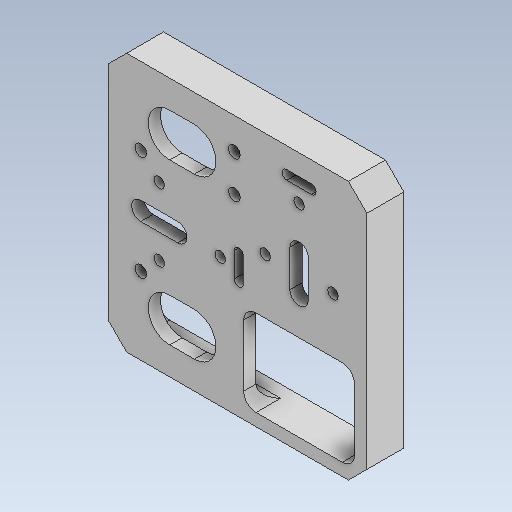
# Autodesk Inventor part: base_shell_1
Saved by Autodesk Inventor 2020 (Build 240168000, 168)
## iProperties
Created: 2022-01-22
Part Number: base_shell_1
Material: Generic
Document SubType Name: Modeling
Designer: Shuang Peng
Density: 1 g/cm^3
Appearance: Default
Author: Shuang Peng
Autodesk Inventor part; units mm, degrees
ref_plane "YZ Plane" through (0, 0, 0) normal (1, 0, 0) x (0, 1, 0)
ref_plane "XZ Plane" through (0, 0, 0) normal (0, 1, 0) x (-1, 0, 0)
ref_plane "XY Plane" through (0, 0, 0) normal (0, 0, 1) x (1, 0, 0)
sketch "Sketch1" plane through (0, 0, 0) normal (0, 0, 1) x (1, 0, 0)
  circle A0 centre (7.5, 4) radius 0.75 projected
  circle A1 centre (13, -5.9) radius 0.75 projected
  circle A2 centre (2, -5.9) radius 0.75 projected
  line L0 (15, -7) -> (15, 0) projected
  line L1 (11, 0) -> (15, 0) projected
  arc A3 (10, 1) -> (11, 0) centre (11, 1) ccw projected
  line L2 (10, 1) -> (10, 5) projected
  line L3 (6, 6) -> (9, 6) projected
  line L4 (5, 1) -> (5, 5) projected
  arc A4 (4, 0) -> (5, 1) centre (4, 1) ccw projected
  line L5 (0, 0) -> (4, 0) projected
  line L6 (0, -7) -> (0, 0) projected
  line L7 (1.5, -8.5) -> (5, -8.5) projected
  line L8 (13, -5.9) -> (2, -5.9)
  line L9 (7.5, -5.9) -> (7.5, -9.9)
  line L10 (7.5, -9.9) -> (-2.5, -9.9)
  line L11 (-23.5, -30.9) -> (-23.5, 11.1)
  line L12 (-23.5, 11.1) -> (18.5, 11.1)
  line L13 (18.5, 11.1) -> (18.5, -30.9)
  line L14 (18.5, -30.9) -> (-23.5, -30.9)
  line L15 (-23.5, -30.9) -> (18.5, 11.1) construction
  line L16 (-23.5, 11.1) -> (18.5, -30.9) construction
  circle A5 centre (-15.2, -15.4) radius 0.75 projected
  circle A6 centre (-15.2, -4.4) radius 0.75 projected
  circle A7 centre (-15.2, -15.4) radius 0.85
  circle A8 centre (-15.2, -4.4) radius 0.85
  circle A9 centre (-5.3, -9.9) radius 0.75 projected
  circle A10 centre (-5.3, -9.9) radius 0.85
  circle A11 centre (2, -5.9) radius 0.85
  circle A12 centre (13, -5.9) radius 0.85
  circle A13 centre (7.5, 4) radius 0.85
  line L17 (6, -7.5) -> (6, -4.5) projected
  arc A14 (9, -4.5) -> (6, -4.5) centre (7.5, -4.5) ccw projected
  line L18 (9, -4.5) -> (9, -7.5) projected
  line L19 (10, -8.5) -> (13.5, -8.5) projected
  arc A15 (6, 6) -> (5, 5) centre (6, 5) ccw projected
  line L20 (1.5, -8.5) -> (0, -7) projected
  arc A16 (5, -8.5) -> (6, -7.5) centre (5, -7.5) ccw projected
  arc A17 (9, -7.5) -> (10, -8.5) centre (10, -7.5) ccw projected
  line L21 (15, -7) -> (13.5, -8.5) projected
  arc A18 (10, 5) -> (9, 6) centre (9, 5) ccw projected
  dimension "d0" = 4
  dimension "d1" = 10
  dimension "d2" = 42
  dimension "d3" = 42
  dimension "d4" = 1.7
  dimension "d5" = 1.7
  dimension "d6" = 1.7
  dimension "d7" = 1.7
  dimension "d8" = 1.7
  dimension "d9" = 1.7
  constraints: 18 end point, 6 centre point, 6 coincident, 3 midpoint, 3 perpendicular, 2 parallel, 1 horizontal, 1 vertical
  measures "d0" distance of L9.start L9.end
  measures "d1" distance of L9.end L10.end
  measures "d2" distance of L11.start L11.end
  measures "d3" distance of L11.end L12.end
  measures "d4" diameter of A7
  measures "d5" diameter of A8
  measures "d6" diameter of A10
  measures "d7" diameter of A11
  measures "d8" diameter of A12
  measures "d9" diameter of A13
extrude "Extrusion1" add sketch "Sketch1" along normal blind 2 contours L21 L19 A17 L18 A14 L17 A16 L7 L20 L6 L5 A4 L4 A15 L3 A18 L2 A3 L1 L0 | L8 L17 A14 L18 | L11 L12 L13 L14
sketch "Sketch2" plane through (0, 0, 0) normal (0, 0, -1) x (-1, 0, 0)
  line L0 (23.5, -30.9) -> (-18.5, -30.9) projected
  line L1 (23.5, 11.1) -> (23.5, -30.9) projected
  line L2 (-18.5, 11.1) -> (23.5, 11.1) projected
  line L3 (-18.5, -30.9) -> (-18.5, 11.1) projected
  circle A0 centre (-2, -5.9) radius 0.85 projected
  circle A1 centre (15.2, -15.4) radius 0.85 projected
  circle A2 centre (15.2, -4.4) radius 0.85 projected
  circle A3 centre (5.3, -9.9) radius 0.85 projected
  circle A4 centre (-13, -5.9) radius 0.85 projected
  circle A5 centre (-7.5, 4) radius 0.85 projected
  line L4 (23.5, -30.9) -> (-18.5, -30.9) projected
  line L5 (-18.5, -30.9) -> (23.5, 11.1)
  line L6 (23.5, -30.9) -> (-18.5, 11.1)
  line L7 (-16.5, -28.9) -> (-16.5, 9.1)
  line L8 (-16.5, 9.1) -> (21.5, 9.1)
  line L9 (21.5, 9.1) -> (21.5, -28.9)
  line L10 (21.5, -28.9) -> (-16.5, -28.9)
  line L11 (-16.5, -28.9) -> (21.5, 9.1) construction
  line L12 (-16.5, 9.1) -> (21.5, -28.9) construction
  point P0 (0, 0)
  point P1 (2.5, -9.9)
  dimension "d12" = 38
  dimension "d13" = 38
  constraints: 16 end point, 3 midpoint, 2 parallel, 1 perpendicular, 1 vertical
  measures "d12" distance of L8.end L9.end
  measures "d13" distance of L7.end L8.end
extrude "Extrusion2" add sketch "Sketch2" along normal blind 4 contours L6 L9 L5 L1 | L0 L5 L10 L6 | L3 L6 L7 L5 | L5 L8 L6 L2
sketch "Sketch3" plane through (0, 0, 2) normal (0, 0, 1) x (1, 0, 0)
  line L0 (16.5, 9.1) -> (16.5, -28.9) projected
  line L1 (16.5, -28.9) -> (-21.5, -28.9) projected
  line L2 (16.5, -28.9) -> (-1.5, -28.9)
  line L3 (-1.5, -28.9) -> (-1.5, -14.9)
  line L4 (-1.5, -14.9) -> (16.5, -14.9)
  line L5 (16.5, -14.9) -> (16.5, -28.9)
  point P0 (0, 0)
  point P1 (-1.5, -28.9)
  dimension "d16" = 18
  dimension "d17" = 14
  constraints: 8 end point, 2 parallel, 1 horizontal, 1 perpendicular
  measures "d16" distance of L3.end L4.end
  measures "d17" distance of L2.end L3.end
extrude "Extrusion3" cut sketch "Sketch3" against normal blind 4
fillet "Fillet1" radius 2 4 edges at (16.5, -14.9, 1) (16.5, -28.9, -1) (-1.5, -28.9, 1) (-1.5, -14.9, 1)
sketch "Sketch4" plane through (-23.5, -30.9, 2) normal (-1, 0, 0) x (0, 0, 1)
  circle A0 centre (-12, 21) radius 0.75 projected
  circle A1 centre (-12, 21) radius 9
  point P0 (-2, 30.9)
  dimension "d21" = 18
  constraints: 1 centre point, 1 coincident
  measures "d21" diameter of A1
extrude "Extrusion4" cut sketch "Sketch4" against normal blind 4
sketch "Sketch5" plane through (0, 0, 0) normal (0, 0, -1) x (-1, 0, 0)
  line L0 (1.5, -16.9) -> (1.5, -26.9) projected
  arc A0 (-0.5, -28.9) -> (1.5, -26.9) centre (-0.5, -26.9) ccw projected
  line L1 (-0.5, -28.9) -> (21.5, -28.9) projected
  line L2 (21.5, -28.9) -> (21.5, 9.1) projected
  line L3 (21.5, 9.1) -> (-16.5, 9.1) projected
  line L4 (-16.5, 9.1) -> (-16.5, -16.9) projected
  arc A1 (-14.5, -14.9) -> (-16.5, -16.9) centre (-14.5, -16.9) ccw projected
  line L5 (-14.5, -14.9) -> (-0.5, -14.9) projected
  arc A2 (1.5, -16.9) -> (-0.5, -14.9) centre (-0.5, -16.9) ccw projected
  circle A3 centre (-2, -5.9) radius 0.85 projected
  circle A4 centre (15.2, -15.4) radius 0.85 projected
  circle A5 centre (15.2, -4.4) radius 0.85 projected
  circle A6 centre (5.3, -9.9) radius 0.85 projected
  circle A7 centre (-13, -5.9) radius 0.85 projected
  circle A8 centre (-7.5, 4) radius 0.85 projected
  line L6 (-7.5, 4) -> (-7.5, 7)
  line L7 (-5.5, 7) -> (-9.5, 7) construction
  line L8 (-5.5, 7.75) -> (-9.5, 7.75)
  line L9 (-9.5, 6.25) -> (-5.5, 6.25)
  arc A9 (-5.5, 6.25) -> (-5.5, 7.75) centre (-5.5, 7) ccw
  arc A10 (-9.5, 7.75) -> (-9.5, 6.25) centre (-9.5, 7) ccw
  line L10 (5.3, -9.9) -> (2.3, -9.9)
  line L11 (2.3, -11.9) -> (2.3, -7.9) construction
  line L12 (3.05, -11.9) -> (3.05, -7.9)
  line L13 (1.55, -7.9) -> (1.55, -11.9)
  arc A11 (1.55, -11.9) -> (3.05, -11.9) centre (2.3, -11.9) ccw
  arc A12 (3.05, -7.9) -> (1.55, -7.9) centre (2.3, -7.9) ccw
  point P0 (0, 0)
  dimension "d24" = 3
  dimension "d25" = 2
  dimension "d26" = 1.5
  dimension "d27" = 3
  dimension "d28" = 2
  dimension "d29" = 1.5
  constraints: 20 end point, 8 point on circle, 8 tangent, 4 centre point, 2 midpoint, 2 parallel, 2 perpendicular, 1 horizontal, 1 vertical
  measures "d24" distance of L6.start L6.end
  measures "d25" distance of L6.end L7.end
  measures "d26" diameter of A10
  measures "d27" distance of L10.start L10.end
  measures "d28" distance of L10.end L11.end
  measures "d29" diameter of A12
extrude "Extrusion5" cut sketch "Sketch5" against normal blind 4 contours A9 L9 A10 L8 | A11 L13 A12 L12
sketch "Sketch6" plane through (0, 0, 0) normal (0, 0, -1) x (-1, 0, 0)
  line L0 (-9.5, 7.75) -> (-5.5, 7.75) projected
  arc A0 (-5.5, 6.25) -> (-5.5, 7.75) centre (-5.5, 7) ccw projected
  line L1 (-5.5, 6.25) -> (-9.5, 6.25) projected
  arc A1 (-9.5, 7.75) -> (-9.5, 6.25) centre (-9.5, 7) ccw projected
  arc A2 (1.55, -11.9) -> (3.05, -11.9) centre (2.3, -11.9) ccw projected
  line L2 (1.55, -11.9) -> (1.55, -7.9) projected
  arc A3 (3.05, -7.9) -> (1.55, -7.9) centre (2.3, -7.9) ccw projected
  line L3 (3.05, -7.9) -> (3.05, -11.9) projected
  line L4 (1.5, -16.9) -> (1.5, -26.9) projected
  arc A4 (-0.5, -28.9) -> (1.5, -26.9) centre (-0.5, -26.9) ccw projected
  line L5 (-0.5, -28.9) -> (21.5, -28.9) projected
  line L6 (21.5, -28.9) -> (21.5, 9.1) projected
  line L7 (21.5, 9.1) -> (-16.5, 9.1) projected
  line L8 (-16.5, 9.1) -> (-16.5, -16.9) projected
  arc A5 (-14.5, -14.9) -> (-16.5, -16.9) centre (-14.5, -16.9) ccw projected
  line L9 (-14.5, -14.9) -> (-0.5, -14.9) projected
  arc A6 (1.5, -16.9) -> (-0.5, -14.9) centre (-0.5, -16.9) ccw projected
  circle A7 centre (-2, -5.9) radius 0.85 projected
  circle A8 centre (15.2, -15.4) radius 0.85 projected
  circle A9 centre (15.2, -4.4) radius 0.85 projected
  circle A10 centre (5.3, -9.9) radius 0.85 projected
  circle A11 centre (-13, -5.9) radius 0.85 projected
  circle A12 centre (-7.5, 4) radius 0.85 projected
  line L10 (15.2, -15.4) -> (15.2, -4.4)
  line L11 (18.2, -9.9) -> (12.2, -9.9) construction
  line L12 (18.2, -8.4) -> (12.2, -8.4)
  line L13 (12.2, -11.4) -> (18.2, -11.4)
  arc A13 (18.2, -11.4) -> (18.2, -8.4) centre (18.2, -9.9) ccw
  arc A14 (12.2, -8.4) -> (12.2, -11.4) centre (12.2, -9.9) ccw
  circle A15 centre (-2, -5.9) radius 0.85 projected
  line L14 (-2, -5.9) -> (-13, -5.9)
  line L15 (-7.5, -8.9) -> (-7.5, -2.9) construction
  line L16 (-6, -8.9) -> (-6, -2.9)
  line L17 (-9, -2.9) -> (-9, -8.9)
  arc A16 (-9, -8.9) -> (-6, -8.9) centre (-7.5, -8.9) ccw
  arc A17 (-6, -2.9) -> (-9, -2.9) centre (-7.5, -2.9) ccw
  point P0 (0, 0)
  point P1 (15.2, -9.9)
  point P2 (-7.5, -5.9)
  dimension "d32" = 3
  dimension "d33" = 3
  dimension "d34" = 3
  dimension "d35" = 3
  constraints: 20 end point, 8 point on circle, 8 tangent, 4 centre point, 4 midpoint, 2 horizontal, 2 parallel, 2 vertical
  measures "d32" distance of point (15.2, -9.9) L11.end
  measures "d33" diameter of A14
  measures "d34" distance of point (-7.5, -5.9) L15.end
  measures "d35" diameter of A17
extrude "Extrusion6" cut sketch "Sketch6" against normal blind 4 contours L13 A14 L12 L10 | L10 L12 A13 L13 | L16 A16 L17 L14 | L14 L17 A17 L16
sketch "Sketch7" plane through (0, 0, 0) normal (0, 0, -1) x (-1, 0, 0)
  line L0 (12.2, -8.4) -> (18.2, -8.4) projected
  arc A0 (18.2, -11.4) -> (18.2, -8.4) centre (18.2, -9.9) ccw projected
  line L1 (18.2, -11.4) -> (12.2, -11.4) projected
  arc A1 (12.2, -8.4) -> (12.2, -11.4) centre (12.2, -9.9) ccw projected
  arc A2 (-9, -8.9) -> (-6, -8.9) centre (-7.5, -8.9) ccw projected
  line L2 (-9, -8.9) -> (-9, -2.9) projected
  arc A3 (-6, -2.9) -> (-9, -2.9) centre (-7.5, -2.9) ccw projected
  line L3 (-6, -2.9) -> (-6, -8.9) projected
  line L4 (-9.5, 7.75) -> (-5.5, 7.75) projected
  arc A4 (-5.5, 6.25) -> (-5.5, 7.75) centre (-5.5, 7) ccw projected
  line L5 (-5.5, 6.25) -> (-9.5, 6.25) projected
  arc A5 (-9.5, 7.75) -> (-9.5, 6.25) centre (-9.5, 7) ccw projected
  arc A6 (1.55, -11.9) -> (3.05, -11.9) centre (2.3, -11.9) ccw projected
  line L6 (1.55, -11.9) -> (1.55, -7.9) projected
  arc A7 (3.05, -7.9) -> (1.55, -7.9) centre (2.3, -7.9) ccw projected
  line L7 (3.05, -7.9) -> (3.05, -11.9) projected
  line L8 (1.5, -16.9) -> (1.5, -26.9) projected
  arc A8 (-0.5, -28.9) -> (1.5, -26.9) centre (-0.5, -26.9) ccw projected
  line L9 (-0.5, -28.9) -> (21.5, -28.9) projected
  line L10 (21.5, -28.9) -> (21.5, 9.1) projected
  line L11 (21.5, 9.1) -> (-16.5, 9.1) projected
  line L12 (-16.5, 9.1) -> (-16.5, -16.9) projected
  arc A9 (-14.5, -14.9) -> (-16.5, -16.9) centre (-14.5, -16.9) ccw projected
  line L13 (-14.5, -14.9) -> (-0.5, -14.9) projected
  arc A10 (1.5, -16.9) -> (-0.5, -14.9) centre (-0.5, -16.9) ccw projected
  circle A11 centre (-2, -5.9) radius 0.85 projected
  circle A12 centre (15.2, -15.4) radius 0.85 projected
  circle A13 centre (15.2, -4.4) radius 0.85 projected
  circle A14 centre (5.3, -9.9) radius 0.85 projected
  circle A15 centre (-13, -5.9) radius 0.85 projected
  circle A16 centre (-7.5, 4) radius 0.85 projected
  line L14 (21.5, -16.6082) -> (21.5, -28.9) projected
  line L15 (21.5, -28.9) -> (21.5, -22.9)
  line L16 (21.5, -22.9) -> (11.5, -22.9)
  line L17 (9.5, -22.9) -> (13.5, -22.9) construction
  line L18 (9.5, -26.4) -> (13.5, -26.4)
  line L19 (13.5, -19.4) -> (9.5, -19.4)
  arc A17 (9.5, -19.4) -> (9.5, -26.4) centre (9.5, -22.9) ccw
  arc A18 (13.5, -26.4) -> (13.5, -19.4) centre (13.5, -22.9) ccw
  line L20 (21.5, 9.1) -> (21.5, 3.1)
  line L21 (21.5, -28.9) -> (21.5, 9.1) projected
  line L22 (21.5, 3.1) -> (11.5, 3.1)
  line L23 (9.5, 3.1) -> (13.5, 3.1) construction
  line L24 (9.5, -0.4) -> (13.5, -0.4)
  line L25 (13.5, 6.6) -> (9.5, 6.6)
  arc A19 (9.5, 6.6) -> (9.5, -0.4) centre (9.5, 3.1) ccw
  arc A20 (13.5, -0.4) -> (13.5, 6.6) centre (13.5, 3.1) ccw
  point P0 (0, 0)
  dimension "d38" = 6
  dimension "d39" = 10
  dimension "d40" = 2
  dimension "d41" = 7
  dimension "d42" = 6
  dimension "d43" = 10
  dimension "d44" = 2
  dimension "d45" = 7
  constraints: 24 end point, 8 point on circle, 8 tangent, 4 centre point, 4 point on line, 2 midpoint, 2 parallel, 1 horizontal, 1 perpendicular
  measures "d38" distance of L9.end L15.end
  measures "d39" distance of L15.end L16.end
  measures "d40" distance of L16.end L17.end
  measures "d41" diameter of A18
  measures "d42" distance of L10.end L20.end
  measures "d43" distance of L20.end L22.end
  measures "d44" distance of L22.end L23.end
  measures "d45" diameter of A20
extrude "Extrusion7" cut sketch "Sketch7" against normal blind 4 contours A17 L19 A18 L18 | A19 L25 A20 L24
fillet "Fillet2" radius 2 3 edges at (16.5, 9.1, -2) (-21.5, 9.1, -2) (-21.5, -28.9, -2)
fillet "Fillet3" radius 2 7 edges at (15.9142, 8.5142, 0) (16.5, -4.9, 0) (-20.9142, 8.5142, 0) (-21.5, -9.9, 0) (-20.9142, -28.3142, 0) (-9.5, -28.9, 0) (-2.5, 9.1, 0)
chamfer "Chamfer1" distance 3 angle 45 4 edges at (-23.5, -30.9, -1) (-23.5, 11.1, -1) (18.5, 11.1, -1) (18.5, -30.9, -1)
sketch "Sketch8" plane through (0, 0, 0) normal (0, 0, -1) x (-1, 0, 0)
  line L0 (19.5, -26.9) -> (1.5, -26.9) projected
  line L1 (19.5, -10.6483) -> (19.5, -26.9) projected
  arc A0 (18.2, -11.4) -> (19.5, -10.6483) centre (18.2, -9.9) ccw projected
  line L2 (18.2, -11.4) -> (12.2, -11.4) projected
  arc A1 (12.2, -8.4) -> (12.2, -11.4) centre (12.2, -9.9) ccw projected
  line L3 (12.2, -8.4) -> (18.2, -8.4) projected
  arc A2 (19.5, -9.1517) -> (18.2, -8.4) centre (18.2, -9.9) ccw projected
  line L4 (19.5, 7.1) -> (19.5, -9.1517) projected
  line L5 (-4.7567, 7.1) -> (19.5, 7.1) projected
  arc A3 (-5.5, 6.25) -> (-4.7567, 7.1) centre (-5.5, 7) ccw projected
  line L6 (-5.5, 6.25) -> (-9.5, 6.25) projected
  arc A4 (-10.2433, 7.1) -> (-9.5, 6.25) centre (-9.5, 7) ccw projected
  line L7 (-14.5, 7.1) -> (-10.2433, 7.1) projected
  line L8 (-14.5, -14.9) -> (-14.5, 7.1) projected
  line L9 (-14.5, -14.9) -> (-0.5, -14.9) projected
  arc A5 (1.5, -16.9) -> (-0.5, -14.9) centre (-0.5, -16.9) ccw projected
  line L10 (1.5, -16.9) -> (1.5, -26.9) projected
  circle A6 centre (-2, -5.9) radius 0.85 projected
  circle A7 centre (15.2, -15.4) radius 0.85 projected
  circle A8 centre (15.2, -4.4) radius 0.85 projected
  circle A9 centre (5.3, -9.9) radius 0.85 projected
  circle A10 centre (-13, -5.9) radius 0.85 projected
  circle A11 centre (-7.5, 4) radius 0.85 projected
  line L11 (1.55, -11.9) -> (1.55, -7.9) projected
  arc A12 (3.05, -7.9) -> (1.55, -7.9) centre (2.3, -7.9) ccw projected
  line L12 (3.05, -7.9) -> (3.05, -11.9) projected
  arc A13 (1.55, -11.9) -> (3.05, -11.9) centre (2.3, -11.9) ccw projected
  line L13 (-6, -2.9) -> (-6, -8.9) projected
  arc A14 (-9, -8.9) -> (-6, -8.9) centre (-7.5, -8.9) ccw projected
  line L14 (-9, -8.9) -> (-9, -2.9) projected
  arc A15 (-6, -2.9) -> (-9, -2.9) centre (-7.5, -2.9) ccw projected
  arc A16 (9.5, -19.4) -> (9.5, -26.4) centre (9.5, -22.9) ccw projected
  line L15 (9.5, -19.4) -> (13.5, -19.4) projected
  arc A17 (13.5, -26.4) -> (13.5, -19.4) centre (13.5, -22.9) ccw projected
  line L16 (13.5, -26.4) -> (9.5, -26.4) projected
  line L17 (13.5, -0.4) -> (9.5, -0.4) projected
  arc A18 (9.5, 6.6) -> (9.5, -0.4) centre (9.5, 3.1) ccw projected
  line L18 (9.5, 6.6) -> (13.5, 6.6) projected
  arc A19 (13.5, -0.4) -> (13.5, 6.6) centre (13.5, 3.1) ccw projected
  line L19 (15.2, -4.4) -> (18.2, -4.4)
  line L20 (18.2, -4.4) -> (18.2, -1.4)
  line L21 (15.2, -15.4) -> (18.2, -15.4)
  line L22 (18.2, -15.4) -> (18.2, -18.4)
  circle A20 centre (18.2, -1.4) radius 0.95
  circle A21 centre (18.2, -18.4) radius 0.95
  point P0 (0, 0)
  dimension "d53" = 3
  dimension "d54" = 3
  dimension "d55" = 3
  dimension "d56" = 3
  dimension "d57" = 1.9
  dimension "d58" = 1.9
  constraints: 8 end point, 2 centre point, 2 coincident, 2 horizontal, 2 perpendicular
  measures "d53" distance of L19.start L19.end
  measures "d54" distance of L19.end L20.end
  measures "d55" distance of L21.start L21.end
  measures "d56" distance of L21.end L22.end
  measures "d57" diameter of A20
  measures "d58" diameter of A21
extrude "Extrusion8" cut sketch "Sketch8" against normal blind 4 contours A20 | A21
sketch "Sketch9" plane through (0, 0, 0) normal (0, 0, -1) x (-1, 0, 0)
  circle A0 centre (18.2, -18.4) radius 0.95 projected
  circle A1 centre (18.2, -1.4) radius 0.95 projected
  line L0 (19.5, -26.9) -> (1.5, -26.9) projected
  line L1 (19.5, -10.6483) -> (19.5, -26.9) projected
  arc A2 (18.2, -11.4) -> (19.5, -10.6483) centre (18.2, -9.9) ccw projected
  line L2 (18.2, -11.4) -> (12.2, -11.4) projected
  arc A3 (12.2, -8.4) -> (12.2, -11.4) centre (12.2, -9.9) ccw projected
  line L3 (12.2, -8.4) -> (18.2, -8.4) projected
  arc A4 (19.5, -9.1517) -> (18.2, -8.4) centre (18.2, -9.9) ccw projected
  line L4 (19.5, 7.1) -> (19.5, -9.1517) projected
  line L5 (-4.7567, 7.1) -> (19.5, 7.1) projected
  arc A5 (-5.5, 6.25) -> (-4.7567, 7.1) centre (-5.5, 7) ccw projected
  line L6 (-5.5, 6.25) -> (-9.5, 6.25) projected
  arc A6 (-10.2433, 7.1) -> (-9.5, 6.25) centre (-9.5, 7) ccw projected
  line L7 (-14.5, 7.1) -> (-10.2433, 7.1) projected
  line L8 (-14.5, -14.9) -> (-14.5, 7.1) projected
  line L9 (-14.5, -14.9) -> (-0.5, -14.9) projected
  arc A7 (1.5, -16.9) -> (-0.5, -14.9) centre (-0.5, -16.9) ccw projected
  line L10 (1.5, -16.9) -> (1.5, -26.9) projected
  circle A8 centre (-2, -5.9) radius 0.85 projected
  circle A9 centre (15.2, -15.4) radius 0.85 projected
  circle A10 centre (15.2, -4.4) radius 0.85 projected
  circle A11 centre (5.3, -9.9) radius 0.85 projected
  circle A12 centre (-13, -5.9) radius 0.85 projected
  circle A13 centre (-7.5, 4) radius 0.85 projected
  line L11 (1.55, -11.9) -> (1.55, -7.9) projected
  arc A14 (3.05, -7.9) -> (1.55, -7.9) centre (2.3, -7.9) ccw projected
  line L12 (3.05, -7.9) -> (3.05, -11.9) projected
  arc A15 (1.55, -11.9) -> (3.05, -11.9) centre (2.3, -11.9) ccw projected
  line L13 (-6, -2.9) -> (-6, -8.9) projected
  arc A16 (-9, -8.9) -> (-6, -8.9) centre (-7.5, -8.9) ccw projected
  line L14 (-9, -8.9) -> (-9, -2.9) projected
  arc A17 (-6, -2.9) -> (-9, -2.9) centre (-7.5, -2.9) ccw projected
  arc A18 (9.5, -19.4) -> (9.5, -26.4) centre (9.5, -22.9) ccw projected
  line L15 (9.5, -19.4) -> (13.5, -19.4) projected
  arc A19 (13.5, -26.4) -> (13.5, -19.4) centre (13.5, -22.9) ccw projected
  line L16 (13.5, -26.4) -> (9.5, -26.4) projected
  line L17 (13.5, -0.4) -> (9.5, -0.4) projected
  arc A20 (9.5, 6.6) -> (9.5, -0.4) centre (9.5, 3.1) ccw projected
  line L18 (9.5, 6.6) -> (13.5, 6.6) projected
  arc A21 (13.5, -0.4) -> (13.5, 6.6) centre (13.5, 3.1) ccw projected
  line L19 (0, 0) -> (3, 0)
  line L20 (3, 0) -> (3, 6)
  circle A22 centre (3, 6) radius 0.95
  circle A23 centre (3, 0) radius 0.95
  dimension "d61" = 3
  dimension "d62" = 6
  dimension "d63" = 1.9
  dimension "d64" = 1.9
  constraints: 4 end point, 2 centre point, 2 coincident, 1 horizontal, 1 vertical
  measures "d61" distance of L19.start L19.end
  measures "d62" distance of L19.end L20.end
  measures "d63" diameter of A22
  measures "d64" diameter of A23
extrude "Extrusion9" cut sketch "Sketch9" against normal blind 4 contours A23 L20 L19 | L19 L20 A23 | A22
sketch "Sketch10" plane through (0, 0, 0) normal (0, 0, -1) x (-1, 0, 0)
  circle A0 centre (3, 0) radius 0.95 projected
  circle A1 centre (3, 6) radius 0.95 projected
  circle A2 centre (18.2, -18.4) radius 0.95 projected
  circle A3 centre (18.2, -1.4) radius 0.95 projected
  line L0 (19.5, -26.9) -> (1.5, -26.9) projected
  line L1 (19.5, -10.6483) -> (19.5, -26.9) projected
  arc A4 (18.2, -11.4) -> (19.5, -10.6483) centre (18.2, -9.9) ccw projected
  line L2 (18.2, -11.4) -> (12.2, -11.4) projected
  arc A5 (12.2, -8.4) -> (12.2, -11.4) centre (12.2, -9.9) ccw projected
  line L3 (12.2, -8.4) -> (18.2, -8.4) projected
  arc A6 (19.5, -9.1517) -> (18.2, -8.4) centre (18.2, -9.9) ccw projected
  line L4 (19.5, 7.1) -> (19.5, -9.1517) projected
  line L5 (-4.7567, 7.1) -> (19.5, 7.1) projected
  arc A7 (-5.5, 6.25) -> (-4.7567, 7.1) centre (-5.5, 7) ccw projected
  line L6 (-5.5, 6.25) -> (-9.5, 6.25) projected
  arc A8 (-10.2433, 7.1) -> (-9.5, 6.25) centre (-9.5, 7) ccw projected
  line L7 (-14.5, 7.1) -> (-10.2433, 7.1) projected
  line L8 (-14.5, -14.9) -> (-14.5, 7.1) projected
  line L9 (-14.5, -14.9) -> (-0.5, -14.9) projected
  arc A9 (1.5, -16.9) -> (-0.5, -14.9) centre (-0.5, -16.9) ccw projected
  line L10 (1.5, -16.9) -> (1.5, -26.9) projected
  circle A10 centre (-2, -5.9) radius 0.85 projected
  circle A11 centre (15.2, -15.4) radius 0.85 projected
  circle A12 centre (15.2, -4.4) radius 0.85 projected
  circle A13 centre (5.3, -9.9) radius 0.85 projected
  circle A14 centre (-13, -5.9) radius 0.85 projected
  circle A15 centre (-7.5, 4) radius 0.85 projected
  line L11 (1.55, -11.9) -> (1.55, -7.9) projected
  arc A16 (3.05, -7.9) -> (1.55, -7.9) centre (2.3, -7.9) ccw projected
  line L12 (3.05, -7.9) -> (3.05, -11.9) projected
  arc A17 (1.55, -11.9) -> (3.05, -11.9) centre (2.3, -11.9) ccw projected
  line L13 (-6, -2.9) -> (-6, -8.9) projected
  arc A18 (-9, -8.9) -> (-6, -8.9) centre (-7.5, -8.9) ccw projected
  line L14 (-9, -8.9) -> (-9, -2.9) projected
  arc A19 (-6, -2.9) -> (-9, -2.9) centre (-7.5, -2.9) ccw projected
  arc A20 (9.5, -19.4) -> (9.5, -26.4) centre (9.5, -22.9) ccw projected
  line L15 (9.5, -19.4) -> (13.5, -19.4) projected
  arc A21 (13.5, -26.4) -> (13.5, -19.4) centre (13.5, -22.9) ccw projected
  line L16 (13.5, -26.4) -> (9.5, -26.4) projected
  line L17 (13.5, -0.4) -> (9.5, -0.4) projected
  arc A22 (9.5, 6.6) -> (9.5, -0.4) centre (9.5, 3.1) ccw projected
  line L18 (9.5, 6.6) -> (13.5, 6.6) projected
  arc A23 (13.5, -0.4) -> (13.5, 6.6) centre (13.5, 3.1) ccw projected
  line L19 (3, 0) -> (3, 6) construction
  line L20 (5.3, 0) -> (5.3, 6)
  line L21 (0.7, 6) -> (0.7, 0)
  arc A24 (0.7, 0) -> (5.3, 0) centre (3, 0) ccw
  arc A25 (5.3, 6) -> (0.7, 6) centre (3, 6) ccw
  line L22 (0.7, 6) -> (5.3, 6)
  line L23 (5.3, 6) -> (5.3, 10)
  line L24 (5.3, 10) -> (0.7, 10)
  line L25 (0.7, 10) -> (0.7, 6)
  point P0 (0, 0)
  point P1 (3, 3)
  dimension "d67" = 4.6
  dimension "d68" = 4.6
  dimension "d69" = 4
  constraints: 16 end point, 4 point on circle, 4 tangent, 3 parallel, 2 centre point, 1 horizontal, 1 midpoint, 1 perpendicular, 1 vertical
  measures "d67" diameter of A25
  measures "d68" distance of L24.end L23.end
  measures "d69" distance of L23.end L22.end
extrude "Extrusion10" add sketch "Sketch10" along normal blind 2.5 contours L22 L20 A24 L21 A1 | A1 L22 A25 L5 | A25 L5 L23 | L25 L5 A25 | A25 L5 L25 L24 L23 | L5 A25
fillet "Fillet4" radius 0.5 8 edges at (-3, 9.1, -2.5) (-5.3, 3.55, 0) (-3, -2.3, 0) (-0.7, 3.55, 0) (-0.7, 8.5142, -0.5858) (-0.7, 9.1, -2.25) (-5.3, 9.1, -2.25) (-5.3, 8.5142, -0.5858)
body "Solid1"
